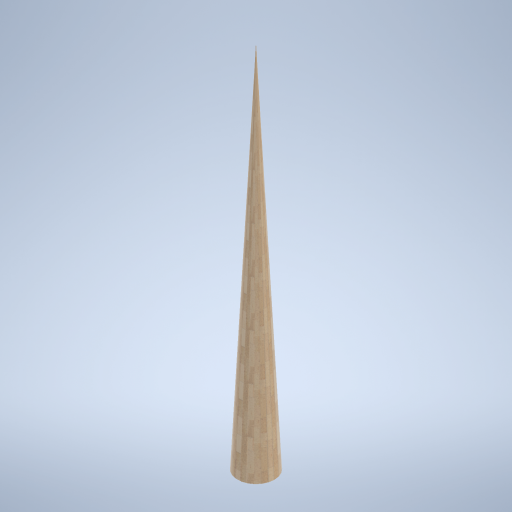
# Autodesk Inventor part: trianglef
Saved by Autodesk Inventor 2023 (Build 270158000, 158)
## iProperties
Created: 2023-10-27
Part Number: trianglef
Material: Wood (Maple)
Document SubType Name: Modeling
Designer: Admin
Density: 0.67 g/cm^3
Appearance: Natural Maple - Glossy Dark Tint
Author: Admin
Autodesk Inventor part; units mm, degrees
ref_plane "YZ Plane" through (0, 0, 0) normal (1, 0, 0) x (0, 1, 0)
ref_plane "XZ Plane" through (0, 0, 0) normal (0, 1, 0) x (-1, 0, 0)
ref_plane "XY Plane" through (0, 0, 0) normal (0, 0, 1) x (1, 0, 0)
sketch "Sketch1" plane through (0, 0, 0) normal (0, 0, 1) x (1, 0, 0)
  line L0 (0, 0) -> (400, 0)
  line L1 (400, 0) -> (0, 8000)
  line L2 (0, 8000) -> (0, 0)
  dimension "d0" = 8000
  dimension "d1" = 400
  dimension "d2" = 8000
  constraints: 6 end point, 1 horizontal, 1 vertical
  measures "d0" vertical distance of L0.end L1.end
  measures "d1" distance of L0.start L0.end
  measures "d2" distance of L1.end L2.end
revolve "Revolution1" add sketch "Sketch1" angle 360 about axis through (0, 8000, 0) along (0, -1, 0)
body "Solid1"
